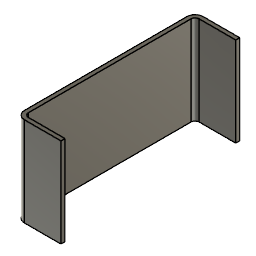
C-200×50×50×4.5 (Autodesk Fusion 360 design; units mm, degrees)
Autodesk Fusion 360 part; units mm, degrees
sketch "スケッチ1" plane through (0, 0, 0) normal (0, 0, 1) x (1, 0, 0)
  line L0 (333.3884, 190.0279) -> (333.3884, 8.0279)
  line L1 (337.8884, 190.0279) -> (337.8884, 8.0279)
  line L2 (342.3884, 3.5279) -> (383.3884, 3.5279)
  line L3 (342.3884, -0.9721) -> (383.3884, -0.9721)
  arc A0 (337.8884, 8.0279) -> (342.3884, 3.5279) centre (342.3884, 8.0279) ccw
  arc A1 (333.3884, 8.0279) -> (342.3884, -0.9721) centre (342.3884, 8.0279) ccw
  line L4 (383.3884, 3.5279) -> (383.3884, -0.9721)
  line L5 (342.3884, 199.0279) -> (383.3884, 199.0279)
  line L6 (342.3884, 194.5279) -> (383.3884, 194.5279)
  arc A2 (342.3884, 194.5279) -> (337.8884, 190.0279) centre (342.3884, 190.0279) ccw
  arc A3 (342.3884, 199.0279) -> (333.3884, 190.0279) centre (342.3884, 190.0279) ccw
  line L7 (383.3884, 199.0279) -> (383.3884, 194.5279)
  point P0 (333.3884, 199.0279)
extrude "押し出し1" add sketch "スケッチ1" along normal blind 100
